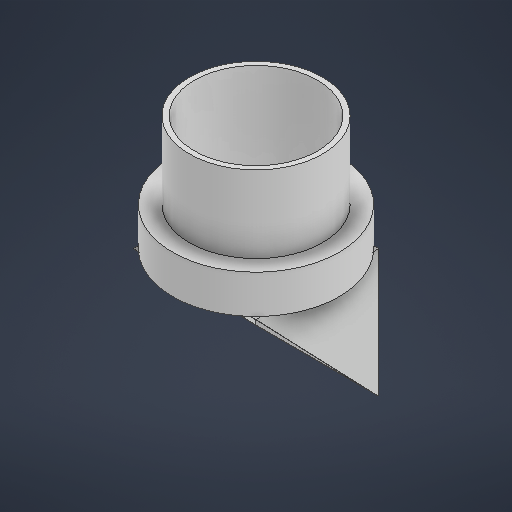
# Autodesk Inventor part: cam_bottom_mount
Saved by Autodesk Inventor 2027 (Build 310192060, 192F)
## iProperties
Created: 2026-07-30
Part Number: cam_bottom_mount
Material: Generic
Document SubType Name: Modeling
Designer: farde
Density: 1 g/cm^3
Appearance: Default
Author: farde
Autodesk Inventor part; units mm, degrees
ref_plane "YZ Plane" through (0, 0, 0) normal (1, 0, 0) x (0, 1, 0)
ref_plane "XZ Plane" through (0, 0, 0) normal (0, 1, 0) x (-1, 0, 0)
ref_plane "XY Plane" through (0, 0, 0) normal (0, 0, 1) x (1, 0, 0)
sketch "Sketch1" plane through (0, 0, 0) normal (0, 1, 0) x (-1, 0, 0)
  circle A0 centre (0, 0) radius 26
  dimension "d0" = 52
  constraints: 1 centre point, 1 coincident
  measures "d0" diameter of A0
extrude "Extrusion1" add sketch "Sketch1" along normal blind 30
sketch "Sketch2" plane through (0, 0, 0) normal (0, -1, 0) x (1, 0, 0)
  circle A0 centre (0, 0) radius 32.5
  dimension "d3" = 65
  constraints: 1 centre point, 1 coincident
  measures "d3" diameter of A0
extrude "Extrusion2" add sketch "Sketch2" along normal blind 15
sketch "Sketch3" plane through (0, 30, 0) normal (0, 1, 0) x (1, 0, 0)
  circle A0 centre (0, 0) radius 24
  dimension "d6" = 48
  constraints: 1 centre point, 1 coincident
  measures "d6" diameter of A0
extrude "Extrusion3" cut sketch "Sketch3" against normal blind 214.475
sketch "Sketch4" plane through (0, -15, 0) normal (0, -1, 0) x (1, 0, 0)
  point P0 (0, 0)
sketch "Sketch7" plane through (0, -15, 0) normal (0, -1, 0) x (1, 0, 0)
  line L0 (24, -24) -> (-24, -24)
  line L1 (-24, -24) -> (-24, 24)
  line L2 (-24, 24) -> (24, 24)
  line L3 (24, 24) -> (24, -24)
  line L4 (24, -24) -> (-24, 24) construction
  line L5 (-24, -24) -> (24, 24) construction
  point P0 (0, 0)
  dimension "d14" = 48
  dimension "d15" = 48
  constraints: 12 end point, 2 midpoint, 2 parallel, 1 horizontal, 1 perpendicular
  measures "d14" distance of L0.end L1.end
  measures "d15" distance of L1.end L2.end
extrude "Extrusion6" add sketch "Sketch7" along normal blind 50
sketch "Sketch8" plane through (0, -65, 0) normal (0, -1, 0) x (1, 0, 0)
  line L0 (-21, 21) -> (21, 21)
  line L1 (21, 21) -> (21, -21)
  line L2 (21, -21) -> (-21, -21)
  line L3 (-21, -21) -> (-21, 21)
  line L4 (-21, 21) -> (21, -21) construction
  line L5 (21, 21) -> (-21, -21) construction
  point P0 (0, 0)
  dimension "d18" = 42
  dimension "d19" = 42
  constraints: 12 end point, 2 midpoint, 2 parallel, 1 horizontal, 1 perpendicular
  measures "d18" distance of L1.end L2.end
  measures "d19" distance of L0.end L1.end
extrude "Extrusion7" cut sketch "Sketch8" against normal blind 47.5
sketch "Sketch9" plane through (24, -15, -21.9146) normal (1, 0, 0) x (0, 0, -1)
  line L0 (2.0854, -50) -> (-45.9146, -50) projected
  line L1 (-45.9146, 0) -> (-45.9146, -50) projected
  line L2 (2.0854, -50) -> (-45.9146, 0)
  line L3 (-45.9146, 0) -> (-45.9146, -50)
  line L4 (-42.9146, -50) -> (-42.9146, -2.5) projected
  line L5 (-45.9146, -50) -> (2.0854, -50)
  point P0 (-21.9146, 15)
  constraints: 6 end point, 1 parallel, 1 perpendicular
extrude "Extrusion8" cut sketch "Sketch9" against normal blind 89.6875
sketch "Sketch10" plane through (0, -17.5, 0) normal (0, -1, 0) x (1, 0, 0)
  circle A0 centre (0, 0) radius 5
  dimension "d24" = 10
  constraints: 1 centre point, 1 coincident
  measures "d24" diameter of A0
extrude "Extrusion9" cut sketch "Sketch10" against normal blind 12.9125
sketch "Sketch11" plane through (-21.9146, -15, -24) normal (0, 0, -1) x (-1, 0, 0)
  circle A0 centre (-21.9146, -24.6875) radius 5
  point P0 (-21.9146, 15)
  dimension "d27" = 10
  constraints: 1 centre point
  measures "d27" diameter of A0
extrude "Extrusion10" cut sketch "Sketch11" against normal blind 74.7375
body "Solid1"
